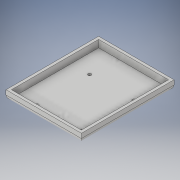
# Autodesk Inventor part: MainPCB_RPI_Top
Saved by Autodesk Inventor 2019.4 (Build 234330000, 330)
## iProperties
Created: 2020-03-12
Part Number: MainPCB_RPI_Top
Material: Generic
Document SubType Name: Modeling
Designer: Jorian Bruslind
Density: 1 g/cm^3
Appearance: Default
Author: Jorian Bruslind
Autodesk Inventor part; units mm, degrees
ref_plane "YZ Plane" through (0, 0, 0) normal (1, 0, 0) x (0, 1, 0)
ref_plane "XZ Plane" through (0, 0, 0) normal (0, 1, 0) x (-1, 0, 0)
ref_plane "XY Plane" through (0, 0, 0) normal (0, 0, 1) x (1, 0, 0)
sketch "Sketch1" plane through (0, 0, 0) normal (0, 1, 0) x (-1, 0, 0)
  line L0 (0, 0) -> (77, 0)
  line L1 (77, 0) -> (77, -96)
  line L2 (77, -96) -> (0, -96)
  line L3 (0, -96) -> (0, 0)
  line L4 (80, -99) -> (80, 3)
  line L5 (80, 3) -> (-3, 3)
  line L6 (-3, 3) -> (-3, -99)
  line L7 (-3, -99) -> (80, -99)
  dimension "d0" = 77
  dimension "d1" = 96
  dimension "d2" = 3
  constraints: 16 end point, 4 parallel, 2 perpendicular, 1 horizontal, 3 other
  measures "d0" distance of L1.end L2.end
  measures "d1" distance of L0.end L1.end
  measures "d2" distance between parallel lines of L1 L4
extrude "Extrusion1" add sketch "Sketch1" along normal blind 10 contours L0 L1 L2 L3 | L7 L6 L5 L4
sketch "Sketch2" plane through (0, 10, 0) normal (0, 1, 0) x (1, 0, 0)
  line L0 (0, 0) -> (-77, 0)
  line L1 (-77, 0) -> (-77, 96)
  line L2 (-77, 96) -> (0, 96)
  line L3 (0, 96) -> (0, 0)
  dimension "d5" = 77
  dimension "d6" = 96
  constraints: 8 end point, 2 parallel, 1 horizontal, 1 perpendicular
  measures "d5" distance of L1.end L2.end
  measures "d6" distance of L0.end L1.end
extrude "Extrusion2" cut sketch "Sketch2" against normal blind 8
sketch "Sketch3" plane through (0, 2, 0) normal (0, 1, 0) x (1, 0, 0)
  line L0 (0, 96) -> (0, 0) projected
  line L1 (0, 0) -> (0, 7.5)
  line L2 (0, 7.5) -> (-7.5, 7.5)
  circle A0 centre (-7.5, 7.5) radius 1.75
  circle A1 centre (-7.5, 65.5) radius 1.75
  circle A2 centre (-56.5, 7.5) radius 1.75
  circle A3 centre (-56.5, 65.5) radius 1.75
  dimension "d9" = 7.5
  dimension "d10" = 7.5
  dimension "d11" = 3.5
  dimension "d14" = 58
  dimension "d17" = 49
  constraints: 4 centre point, 4 end point, 1 coincident, 1 horizontal, 1 perpendicular, 1 point on line, 1 vertical, 6 other
  measures "d9" distance of L0.end L1.end
  measures "d10" distance of L1.end L2.end
  measures "d11" diameter of A0
  measures "d14" distance of A0.centre A1.centre
  measures "d17" distance of A0.centre A2.centre
extrude "Extrusion3" cut sketch "Sketch3" against normal blind 3
fillet "Fillet1" radius 5 4 edges at (-38.5, 0, 3) (-80, 0, -48) (3, 0, -48) (-38.5, 0, -99)
body "Solid1"
